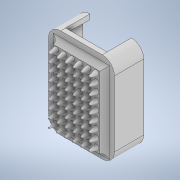
# Autodesk Inventor part: Mold_equalSpacing_2mm
Saved by Autodesk Inventor 2021 (Build 250183000, 183)
## iProperties
Created: 2021-04-08
Part Number: Mold_equalSpacing_2mm
Material: Generic
Document SubType Name: Modeling
Designer: Olivi
Density: 1 g/cm^3
Appearance: Default
Author: Olivi
Autodesk Inventor part; units mm, degrees
ref_plane "YZ Plane" through (0, 0, 0) normal (1, 0, 0) x (0, 1, 0)
sketch "Sketch1" plane through (0, 0, 0) normal (0, 0, 1) x (1, 0, 0)
  line L0 (0, 0) -> (19.1, 0)
  line L1 (19.1, 0) -> (19.1, 29.4)
  line L2 (19.1, 29.4) -> (0, 29.4)
  line L3 (0, 29.4) -> (0, 0)
  dimension "d0" = 19.1
  dimension "d1" = 29.4
  constraints: 8 end point, 2 horizontal, 2 perpendicular
  measures "d0" distance of L0.start L0.end
  measures "d1" distance of L0.end L1.end
extrude "Extrusion1" add sketch "Sketch1" along normal blind 2
sketch "Sketch2" plane through (0, 0, 2) normal (0, 0, 1) x (1, 0, 0)
  line L0 (0, 29.4) -> (0, 0) projected
  circle A0 centre (1.2, 28.2) radius 1
  line L1 (19.1, 29.4) -> (0, 29.4) projected
  dimension "d6" = 2
  dimension "d7" = 1.2
  dimension "d8" = 1.2
  constraints: 1 centre point
  measures "d6" diameter of A0
  measures "d7" distance from line of L0 A0.centre
  measures "d8" distance from line of L1 A0.centre
ref_plane "Work Plane1" through (0, 0, 5) normal (0, 0, 1) x (1, 0, 0)
ref_plane "Work Plane2" through (0, 0, 4.5) normal (0, 0, 1) x (1, 0, 0)
extrude "Extrusion3" add sketch "Sketch2" along normal blind 3 draft -14
pattern_linear "Rectangular Pattern1" count 6 spacing 3.3 along (1, 0, 0) count 9 spacing 3.3 along (0, -1, 0) of "Extrusion3"
sketch "Sketch6" plane through (0, 0, 0) normal (0, 0, -1) x (-1, 0, 0)
  line L0 (0, 29.4) -> (0, 0) projected
  line L1 (0, 15.2241) -> (0, -3.2759)
  line L2 (0, -3.2759) -> (-19.1, -3.2759)
  line L3 (-19.1, 0) -> (-19.1, 29.4) projected
  line L4 (-19.1, -3.2759) -> (-19.1, 33.7241)
  line L5 (-19.1, 33.7241) -> (0, 33.7241)
  line L6 (0, 33.7241) -> (0, -3.2759)
  line L7 (-9.55, -3.2759) -> (3.95, -3.2759)
  line L8 (3.95, -3.2759) -> (3.95, 33.7241)
  line L9 (3.95, 33.7241) -> (-23.05, 33.7241)
  line L10 (-23.05, 33.7241) -> (-23.05, -3.2759)
  line L11 (-23.05, -3.2759) -> (-19.1, -3.2759)
  dimension "d41" = 13.5
  dimension "d42" = 27
  constraints: 20 end point, 4 perpendicular, 3 point on line, 2 collinear, 1 horizontal, 1 midpoint, 1 vertical
  measures "d41" distance of L7.start L7.end
  measures "d42" distance of L8.end L9.end
extrude "Extrusion4" add sketch "Sketch6" along normal blind 2
fillet "Fillet3" radius 5 4 edges at (23.05, -3.2759, -1) (-3.95, -3.2759, -1) (23.05, 33.7241, -1) (-3.95, 33.7241, -1)
sketch "Sketch8" plane through (0, 0, -2) normal (0, 0, -1) x (-1, 0, 0)
  line L0 (3.95, 1.7241) -> (3.95, 28.7241) projected
  line L1 (3.95, 28.7241) -> (1.95, 28.7241)
  line L2 (1.95, 28.7241) -> (1.95, 1.7241)
  arc A0 (-1.05, -3.2759) -> (3.95, 1.7241) centre (-1.05, 1.7241) ccw projected
  line L3 (1.95, 1.7241) -> (3.95, 1.7241)
  line L4 (3.95, 1.7241) -> (3.95, 28.7241)
  line L5 (-23.05, 28.7241) -> (-23.05, 1.7241) projected
  line L6 (-23.05, 28.7241) -> (-21.05, 28.7241)
  line L7 (-21.05, 28.7241) -> (-21.05, 1.7241)
  line L8 (-21.05, 1.7241) -> (-23.05, 1.7241)
  line L9 (-23.05, 1.7241) -> (-23.05, 28.7241)
  line L10 (1.95, 15) -> (1.95, 14)
  line L11 (1.95, 14) -> (-21.05, 14)
  line L12 (-21.05, 14) -> (-21.05, 16)
  line L13 (-21.05, 16) -> (1.95, 16)
  line L14 (1.95, 15) -> (1.95, 16)
  line L15 (-18.05, -3.2759) -> (-1.05, -3.2759) projected
  line L16 (3.95, 1.7241) -> (3.95, 28.7241) projected
  arc A1 (-1.05, -3.2759) -> (3.95, 1.7241) centre (-1.05, 1.7241) ccw
  line L17 (-1.05, -3.2759) -> (-1.05, -1.2759)
  arc A2 (-1.05, -1.2759) -> (1.95, 1.7241) centre (-1.8843, 2.5584) ccw
  arc A3 (3.95, 28.7241) -> (-1.05, 33.7241) centre (-1.05, 28.7241) ccw projected
  arc A4 (3.95, 28.7241) -> (-1.05, 33.7241) centre (-1.05, 28.7241) ccw
  line L18 (-1.05, 33.7241) -> (-1.05, 31.7241)
  arc A5 (1.95, 28.7241) -> (-1.05, 31.7241) centre (-0.812, 28.962) ccw
  arc A6 (-18.05, 33.7241) -> (-23.05, 28.7241) centre (-18.05, 28.7241) ccw projected
  arc A7 (-18.05, 33.7241) -> (-23.05, 28.7241) centre (-18.05, 28.7241) ccw
  line L19 (-1.05, 33.7241) -> (-18.05, 33.7241) projected
  line L20 (-18.05, 33.7241) -> (-18.05, 31.7241)
  arc A8 (-18.05, 31.7241) -> (-21.05, 28.7241) centre (-18.05, 28.7241) ccw
  arc A9 (-23.05, 1.7241) -> (-18.05, -3.2759) centre (-18.05, 1.7241) ccw
  line L21 (-18.05, -3.2759) -> (-18.05, -1.2759)
  arc A10 (-21.05, 1.7241) -> (-18.05, -1.2759) centre (-17.2612, 2.5129) ccw
  point P0 (0, 0)
  dimension "d48" = 2
  dimension "d49" = 2
  dimension "d50" = 2
  dimension "d53" = 2
  dimension "d54" = 2
  dimension "d55" = 2
  constraints: 34 end point, 16 point on circle, 9 perpendicular, 8 centre point, 7 point on line, 5 tangent, 4 vertical, 1 concentric, 1 horizontal
  measures "d48" distance of L0.end L1.end
  measures "d49" distance of L5.start L6.end
  measures "d50" distance of L11.end L12.end
  measures "d53" distance of L15.end L17.end
  measures "d54" distance of L18.start L18.end
  measures "d55" distance of L19.end L20.end
extrude "Extrusion5" add sketch "Sketch8" along normal blind 10 contours L3 L2 L1 L0 | A0 L17 A2 L3 | L1 A5 L18 A3 | A9 L8 A10 L21 | L11 L7 L13 L2 | L20 A8 L6 A6 | L5 L6 L7 L8
fillet "Fillet4" radius 2 4 edges at (19.1, 14.7, 0) (9.55, 29.4, 0) (0, 14.7, 0) (9.55, 0, 0)
body "Solid1"
